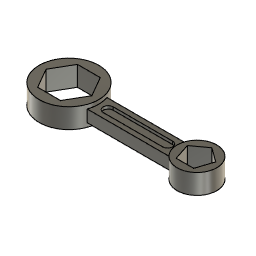
Exercise2 (Autodesk Fusion 360 design; units mm, degrees)
Autodesk Fusion 360 part; units mm, degrees
sketch "Sketch1" plane through (0, 0, 0) normal (0, 0, 1) x (1, 0, 0) in component "Exercise 2"
  circle A0 centre (0, 0) radius 30
  line L0 (30, 0) -> (109, 0) construction
  circle A1 centre (129, 0) radius 20
  line L1 (-23.094, 0) -> (-11.547, -20)
  line L2 (-11.547, -20) -> (11.547, -20)
  line L3 (11.547, -20) -> (23.094, 0)
  line L4 (23.094, 0) -> (11.547, 20)
  line L5 (11.547, 20) -> (-11.547, 20)
  line L6 (-11.547, 20) -> (-23.094, 0)
  line L7 (129, 15) -> (114.7342, 4.6353)
  line L8 (114.7342, 4.6353) -> (120.1832, -12.1353)
  line L9 (120.1832, -12.1353) -> (137.8168, -12.1353)
  line L10 (137.8168, -12.1353) -> (143.2658, 4.6353)
  line L11 (143.2658, 4.6353) -> (129, 15)
  line L12 (28.2843, 10) -> (111.6795, 10)
  line L13 (28.2843, -10) -> (111.6795, -10)
  line L14 (41.522, 10) -> (41.522, -10) construction
  line L15 (41.522, 0) -> (50, 0) construction
  line L16 (69.5, 0) -> (69.5, 26.8283) construction
  line L17 (99.5, 5) -> (39.5, 5)
  line L18 (39.5, -5) -> (99.5, -5)
  line L19 (99.5, 5) -> (39.5, -5) construction
  line L20 (39.5, 5) -> (99.5, -5) construction
  arc A2 (41.522, 4.5729) -> (41.522, -4.5729) centre (39.5, 0) ccw
  arc A3 (97.8784, -4.7297) -> (97.8784, 4.7297) centre (99.5, 0) ccw
  point P0 (129, 0)
  point P1 (69.5, 0)
  dimension "d13" = 60
  dimension "d14" = 129
  dimension "d15" = 40
  dimension "d17" = 20
  dimension "d18" = 15
  dimension "d19" = 20
  dimension "d20" = 60
  dimension "d21" = 10
  dimension "d22" = 10
  constraint coincident A0.centre origin
  constraint horizontal L0
  constraint coincident P0 A1.centre
  constraint horizontal L12
  constraint horizontal L13
  constraint coincident L12 L14.start
  constraint coincident L13 L14.end
  constraint perpendicular L13 L14
  constraint midpoint L14 L15.start
  constraint perpendicular L14 L15
  constraint collinear L0 L15
  constraint coincident A0 L12.start
  constraint coincident A0 L13.start
  constraint coincident A1 L13.end
  constraint coincident A1 L12.end
  constraint coincident A0 L0.start
  constraint coincident A1 L0.end
  constraint midpoint L0 P1
  constraint vertical L16
  constraint horizontal L17
  constraint parallel L17 L18
  constraint coincident L19 P1
  constraint coincident L20 P1
  constraint coincident P1 L16.start
  constraint coincident L17.end A2
  constraint tangent L17 A2
  constraint coincident L18.start A2
  constraint coincident L17.start A3
  constraint tangent L17 A3
  constraint coincident L18.end A3
  constraint coincident L14 A2.start
  constraint coincident L14 A2.end
  constraint coincident L19 A3.end
  constraint coincident L20 A3.start
  measures "d13" diameter of A0
  measures "d14" distance of A0.centre A1.centre
  measures "d15" diameter of A1
  measures "d17" distance of A0.centre L5
  measures "d18" distance of L7.start P0
  measures "d19" distance of L12 L13
  measures "d20" distance of L18.start L18.end
  measures "d21" distance of L17.end L18.start
  measures "d22" distance of L17 L18
extrude "Extrude1" add sketch "Sketch1" along normal mid plane 20 contours A0 | A1 makes body 1 at (27.1662, -12.7278, 3.3333) makes body 2 at (148.9006, -1.9914, -3.3333) in component "Exercise 2"
extrude "Extrude2" add sketch "Sketch1" along normal mid plane 12 contours A0 A1 L12 L13 bodies 1 2 in component "Exercise 2"
extrude "Extrude3" add sketch "Sketch1" along normal mid plane 6 contours L17 L18 A2 A3 bodies 1 in component "Exercise 2"
component "Exercise 2" placed x (1, 0, 0) y (0, 1, 0) z (0, 0, 1) at (0, 0, 0)
